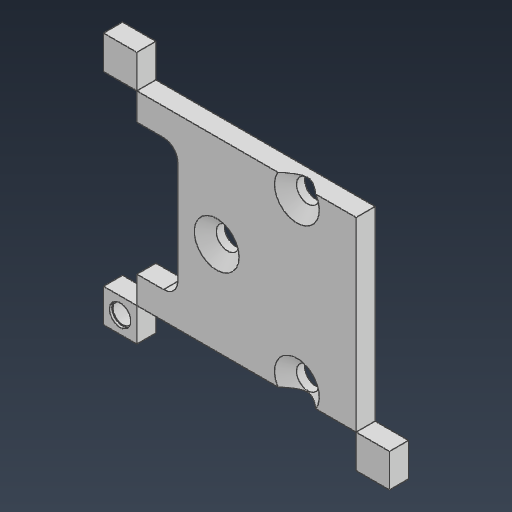
# Autodesk Inventor part: vesc_holder
Saved by Autodesk Inventor 2023 (Build 270158000, 158)
## iProperties
Created: 2026-01-23
Part Number: vesc_holder
Material: Generic
Document SubType Name: Modeling
Designer: szymo
Density: 1 g/cm^3
Appearance: Default
Author: szymo
Autodesk Inventor part; units mm, degrees
ref_plane "YZ Plane" through (0, 0, 0) normal (1, 0, 0) x (0, 1, 0)
ref_plane "XZ Plane" through (0, 0, 0) normal (0, 1, 0) x (-1, 0, 0)
ref_plane "XY Plane" through (0, 0, 0) normal (0, 0, 1) x (1, 0, 0)
sketch "Sketch1" plane through (0, 0, 0) normal (0, 0, 1) x (1, 0, 0)
  circle A0 centre (60.075, 53.025) radius 1.621 projected
  circle A1 centre (43.25, 70) radius 1.621 projected
  circle A2 centre (60.075, 86.975) radius 1.621 projected
  line L0 (72.5, 89.5) -> (26.5, 89.5) projected
  line L1 (26.5, 89.5) -> (26.5, 83.8) projected
  line L2 (26.5, 83.8) -> (32.1, 83.8) projected
  arc A3 (35.1, 80.8) -> (32.1, 83.8) centre (32.1, 80.8) ccw projected
  line L3 (35.1, 80.8) -> (35.1, 59.2) projected
  arc A4 (32.1, 56.2) -> (35.1, 59.2) centre (32.1, 59.2) ccw projected
  line L4 (32.1, 56.2) -> (26.5, 56.2) projected
  line L5 (26.5, 56.2) -> (26.5, 50.5) projected
  line L6 (26.5, 50.5) -> (72.5, 50.5) projected
  line L7 (72.5, 50.5) -> (72.5, 89.5) projected
  circle A5 centre (29.5, 87) radius 1.25 projected
  circle A6 centre (29.5, 53) radius 1.25 projected
  circle A7 centre (69.5, 53) radius 1.25 projected
  circle A8 centre (69.5, 87) radius 1.25 projected
  line L8 (72.5, 89.5) -> (26.5, 89.5)
  line L9 (26.5, 89.5) -> (26.5, 50.5)
  line L10 (26.5, 50.5) -> (72.5, 50.5)
  line L11 (72.5, 50.5) -> (72.5, 89.5)
  point P0 (0, 0)
  point P1 (-13.8, 43.5)
  point P2 (13.8, 43.5)
  constraints: 8 end point, 2 parallel, 1 horizontal, 1 perpendicular
extrude "Extrusion1" add sketch "Sketch1" along normal blind 4 contours A0 | A1 | A2 | L7 L6 L5 L4 A4 L3 A3 L2 L1 L0 | A5 | A6 | A7 | A8
sketch "Sketch2" plane through (0, 0, 4) normal (0, 0, 1) x (1, 0, 0)
  circle A0 centre (60.075, 53.025) radius 1.621 projected
  circle A1 centre (43.25, 70) radius 1.621 projected
  circle A2 centre (60.075, 86.975) radius 1.621 projected
  line L0 (72.5, 89.5) -> (26.5, 89.5) projected
  line L1 (26.5, 89.5) -> (26.5, 83.8) projected
  line L2 (26.5, 83.8) -> (32.1, 83.8) projected
  arc A3 (35.1, 80.8) -> (32.1, 83.8) centre (32.1, 80.8) ccw projected
  line L3 (35.1, 80.8) -> (35.1, 59.2) projected
  arc A4 (32.1, 56.2) -> (35.1, 59.2) centre (32.1, 59.2) ccw projected
  line L4 (32.1, 56.2) -> (26.5, 56.2) projected
  line L5 (26.5, 56.2) -> (26.5, 50.5) projected
  line L6 (26.5, 50.5) -> (72.5, 50.5) projected
  line L7 (72.5, 50.5) -> (72.5, 89.5) projected
  circle A5 centre (29.5, 87) radius 1.25 projected
  circle A6 centre (29.5, 53) radius 1.25 projected
  circle A7 centre (69.5, 53) radius 1.25 projected
  circle A8 centre (69.5, 87) radius 1.25 projected
  point P0 (0, 0)
  constraints: 3 coincident
hole "Hole1" at (60.075, 86.975, 4) at (60.075, 53.025, 4) at (43.25, 70, 4) direction (0, 0, -1) diameter 4.8 depth 5 countersink diameter 9.4 countersink angle 90 clearance for "Countersunk Flat Head Screw ISO 2009/7046" size "M4" standard "ISO"
sketch "Sketch3" plane through (0, 0, 0) normal (0, 0, -1) x (-1, 0, 0)
  line L0 (-64.0391, 50.5) -> (-72.5, 50.5) projected
  line L1 (-72.5, 50.5) -> (-72.5, 89.5) projected
  line L2 (-72.5, 89.5) -> (-64.0391, 89.5) projected
  line L3 (-72.5, 50.5) -> (-72.5, 89.5) projected
  line L4 (-72.5, 89.5) -> (-65.5, 89.5)
  line L5 (-65.5, 89.5) -> (-65.5, 82.5)
  line L6 (-65.5, 82.5) -> (-72.5, 82.5)
  line L7 (-72.5, 82.5) -> (-72.5, 89.5)
  line L8 (-72.5, 50.5) -> (-79.5, 50.5)
  line L9 (-79.5, 50.5) -> (-79.5, 43.5)
  line L10 (-79.5, 43.5) -> (-72.5, 43.5)
  line L11 (-72.5, 43.5) -> (-72.5, 50.5)
  line L12 (-26.5, 89.5) -> (-19.5, 89.5)
  line L13 (-19.5, 89.5) -> (-19.5, 96.5)
  line L14 (-19.5, 96.5) -> (-26.5, 96.5)
  line L15 (-26.5, 96.5) -> (-26.5, 89.5)
  line L16 (-19.5, 50.5) -> (-26.5, 50.5)
  line L17 (-26.5, 50.5) -> (-26.5, 43.5)
  line L18 (-26.5, 43.5) -> (-19.5, 43.5)
  line L19 (-19.5, 43.5) -> (-19.5, 50.5)
  line L20 (-35.1, 80.8) -> (-35.1, 59.2) projected
  arc A0 (-35.1, 59.2) -> (-32.1, 56.2) centre (-32.1, 59.2) ccw projected
  line L21 (-32.1, 56.2) -> (-26.5, 56.2) projected
  line L22 (-26.5, 56.2) -> (-26.5, 50.5) projected
  line L23 (-26.5, 89.5) -> (-26.5, 83.8) projected
  line L24 (-26.5, 83.8) -> (-32.1, 83.8) projected
  arc A1 (-32.1, 83.8) -> (-35.1, 80.8) centre (-32.1, 80.8) ccw projected
  arc A2 (-56.1109, 50.5) -> (-64.0391, 50.5) centre (-60.075, 53.025) ccw projected
  arc A3 (-64.0391, 89.5) -> (-56.1109, 89.5) centre (-60.075, 86.975) ccw projected
  line L25 (-56.1109, 89.5) -> (-26.5, 89.5) projected
  line L26 (-26.5, 50.5) -> (-56.1109, 50.5) projected
  point P0 (0, 0)
  point P1 (-19.5, 82.5)
  point P2 (19.5, 82.5)
  dimension "d9" = 7
  dimension "d10" = 7
  dimension "d11" = 7
  dimension "d12" = 7
  dimension "d15" = 7
  dimension "d16" = 7
  dimension "d17" = 7
  dimension "d18" = 7
  constraints: 32 end point, 8 parallel, 4 horizontal, 4 perpendicular
  measures "d9" distance of L5.end L6.end
  measures "d10" distance of L4.end L5.end
  measures "d11" distance of L10.end L9.end
  measures "d12" distance of L9.end L8.end
  measures "d15" distance of L14.end L13.end
  measures "d16" distance of L13.end L12.end
  measures "d17" distance of L18.end L17.end
  measures "d18" distance of L17.end L16.end
extrude "Extrusion2" add sketch "Sketch3" against normal up to surface (4 mm away) contours L11 L10 L9 L8 | L15 L14 L13 L12 | L16 L19 L18 L17 | L1 L2 L5 L6
sketch "Sketch4" plane through (0, 0, 4) normal (0, 0, -1) x (-1, 0, 0)
  line L0 (-19.5, 89.5) -> (-19.5, 96.5) projected
  line L1 (-19.5, 96.5) -> (-26.5, 96.5) projected
  line L2 (-72.5, 89.5) -> (-26.5, 89.5) projected
  line L3 (-79.5, 50.5) -> (-79.5, 43.5) projected
  line L4 (-79.5, 43.5) -> (-72.5, 43.5) projected
  line L5 (-26.5, 50.5) -> (-72.5, 50.5) projected
  line L6 (-19.5, 50.5) -> (-26.5, 50.5) projected
  line L7 (-26.5, 50.5) -> (-26.5, 43.5) projected
  line L8 (-19.5, 96.5) -> (33.5, 149.5)
  line L9 (19.5, 89.5) -> (-26.5, 89.5) projected
  line L10 (-19.5, 89.5) -> (19.5, 50.5)
  line L11 (-26.5, 50.5) -> (-26.5, 43.5) projected
  line L12 (-26.5, 50.5) -> (-19.5, 43.5)
  line L13 (-26.5, 43.5) -> (-19.5, 50.5)
  line L14 (26.5, 89.5) -> (19.5, 82.5)
  line L15 (28.2348, 94.1586) -> (19.5, 89.5)
  line L16 (-19.5, 50.5) -> (-72.5, 50.5) projected
  line L17 (-79.5, 50.5) -> (-19.5, 82.5)
  line L18 (-19.5, 82.5) -> (-79.5, 82.5)
  line L19 (-79.5, 43.5) -> (-99.5766, 81.1436)
  line L20 (-72.5, 50.5) -> (-72.5, 89.5) projected
  line L21 (-26.5, 56.2) -> (-26.5, 50.5) projected
  line L22 (-32.1, 56.2) -> (-26.5, 56.2) projected
  arc A0 (-35.1, 59.2) -> (-32.1, 56.2) centre (-32.1, 59.2) ccw projected
  line L23 (-35.1, 80.8) -> (-35.1, 59.2) projected
  arc A1 (-32.1, 83.8) -> (-35.1, 80.8) centre (-32.1, 80.8) ccw projected
  line L24 (-26.5, 83.8) -> (-32.1, 83.8) projected
  line L25 (-26.5, 89.5) -> (-26.5, 83.8) projected
  line L26 (-26.5, 43.5) -> (-19.5, 43.5) projected
  line L27 (-19.5, 43.5) -> (-19.5, 50.5) projected
  line L28 (-26.5, 96.5) -> (-26.5, 89.5) projected
  line L29 (-26.5, 89.5) -> (-19.5, 89.5) projected
  line L30 (-72.5, 43.5) -> (-72.5, 50.5) projected
  line L31 (-72.5, 50.5) -> (-79.5, 50.5) projected
  point P0 (0, 0)
  point P1 (-56.1109, 89.5)
  point P2 (-64.0391, 50.5)
  point P3 (0, 70)
  point P4 (-23, 47)
  point P5 (-82.4066, 48.9498)
  point P6 (23.8674, 91.8293)
  constraints: 18 end point, 3 midpoint, 3 perpendicular, 3 point on line, 2 parallel, 1 horizontal, 2 other
hole "Hole2" at (0, 70, 4) at (23, 47, 4) at (82.4066, 48.9498, 4) at (-23.8674, 91.8293, 4) direction (0, 0, -1) diameter 4 depth 5.5 counterbore diameter 4.5 counterbore depth 0.5
body "Solid1"
